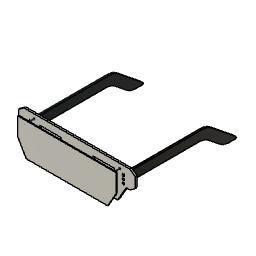
HyperShades mk.2 (Autodesk Fusion 360 design; units mm, degrees)
Autodesk Fusion 360 part; units mm, degrees
sketch "DiffSketch" plane through (0, 0, 0) normal (0, 1, 0) x (1, 0, 0)
  line L0 (-69.215, 0) -> (69.215, 0)
  line L1 (-69.215, 0) -> (-69.215, 25.4)
  line L2 (69.215, 0) -> (69.215, 25.4)
  line L3 (69.215, 25.4) -> (57.1899, 46.228)
  line L4 (57.1899, 46.228) -> (-0.1294, 46.228)
  line L5 (-69.215, 25.4) -> (-57.1899, 46.228)
  line L6 (-57.1899, 46.228) -> (-0.1294, 46.228)
  dimension "d1" = 138.43
  dimension "d3" = 25.4
  dimension "d4" = 25.4
  dimension "d5" = 150
  dimension "d6" = 150
  dimension "d26" = 46.228
  constraint horizontal L0
  constraint coincident origin L0
  constraint perpendicular L0 L1
  constraint perpendicular L0 L2
  constraint coincident L0 origin
  constraint midpoint L0 origin
  constraint horizontal L4
  constraint horizontal L6
  measures "d1" distance of L0.start L0.end
  measures "d3" distance of L0.start L1.end
  measures "d4" distance of L0.end L2.end
  measures "d5" angle of L2 L3
  measures "d6" angle of L1 L5
  measures "d26" vertical distance of origin L4.end
extrude "Extrude1" add sketch "DiffSketch" along normal blind 1.27 makes body 1
sketch "StandSketch" plane through (0, 1.27, 0) normal (0, 1, 0) x (-1, 0, 0)
  line L0 (69.215, 0) -> (-69.215, 0)
  line L1 (-69.215, 0) -> (-69.215, -25.4)
  line L2 (-69.215, -25.4) -> (-57.1899, -46.228)
  line L3 (-57.1899, -46.228) -> (57.1899, -46.228)
  line L4 (57.1899, -46.228) -> (69.215, -25.4)
  line L5 (69.215, -25.4) -> (69.215, 0)
  circle A0 centre (-60.325, -6.35) radius 1.016
  line L6 (-69.215, 0) -> (-60.325, 0) construction
  line L7 (-60.325, 0) -> (-60.325, -6.35) construction
  line L8 (-60.325, -6.35) -> (-69.215, -6.35) construction
  line L9 (-69.215, -6.35) -> (-69.215, 0) construction
  line L10 (69.215, 0) -> (60.325, 0) construction
  line L11 (60.325, 0) -> (60.325, -6.35) construction
  line L12 (60.325, -6.35) -> (69.215, -6.35) construction
  line L13 (69.215, -6.35) -> (69.215, 0) construction
  circle A1 centre (60.325, -6.35) radius 1.016
  line L14 (0, -46.228) -> (-12.7, -46.228) construction
  line L15 (-12.7, -46.228) -> (-12.7, -30.988) construction
  line L16 (-12.7, -30.988) -> (0, -30.988) construction
  line L17 (0, -30.988) -> (0, -46.228) construction
  line L18 (0, -46.228) -> (12.7, -46.228) construction
  line L19 (12.7, -46.228) -> (12.7, -30.988) construction
  line L20 (12.7, -30.988) -> (0, -30.988) construction
  line L21 (0, -30.988) -> (0, -46.228) construction
  circle A2 centre (-12.7, -30.988) radius 1.016
  circle A3 centre (12.7, -30.988) radius 1.016
  dimension "d10" = 2.032
  dimension "d11" = 8.89
  dimension "d12" = 6.35
  dimension "d23" = 8.89
  dimension "d24" = 6.35
  dimension "d25" = 2.032
  dimension "d27" = 12.7
  dimension "d28" = 15.24
  dimension "d29" = 12.7
  dimension "d30" = 15.24
  dimension "d31" = 2.032
  dimension "d32" = 2.032
  constraint horizontal L6
  constraint vertical L7
  constraint horizontal L8
  constraint vertical L9
  constraint coincident L0.end L1.start
  constraint coincident A0.centre L7.end
  constraint horizontal L10
  constraint vertical L11
  constraint horizontal L12
  constraint vertical L13
  constraint coincident L0.start L5.end
  constraint coincident L11.end L12.start
  constraint horizontal L14
  constraint vertical L15
  constraint horizontal L16
  constraint vertical L17
  constraint midpoint L3 L14.start
  constraint horizontal L18
  constraint vertical L19
  constraint horizontal L20
  constraint vertical L21
  constraint coincident L15.end L16.start
  constraint coincident L19.end L20.start
  measures "d10" diameter of A0
  measures "d11" distance of L0.end L6.end
  measures "d12" distance of L0.end L8.end
  measures "d23" distance of L0.start L10.end
  measures "d24" distance of L0.start L12.end
  measures "d25" diameter of A1
  measures "d27" distance of L14.start L14.end
  measures "d28" distance of L14.start L16.end
  measures "d29" distance of L14.start L18.end
  measures "d30" distance of L14.start L16.end
  measures "d31" diameter of A2
  measures "d32" diameter of A3
extrude "Extrude2" add sketch "StandSketch" along normal blind 12.7 separate body contours A0 | A1 | A2 | A3 makes body 2 at (60.3503, 9.7367, -5.3343) makes body 3 at (-60.2997, 9.7367, -5.3343) makes body 4 at (13.4783, 9.7367, -31.6411) makes body 5 at (-11.9217, 9.7367, -31.6411)
sketch "GlassSketch" plane through (0, 13.97, 0) normal (0, 1, 0) x (-1, 0, 0)
  circle A0 centre (-60.325, -6.35) radius 1.016
  line L0 (69.215, 0) -> (-69.215, 0)
  line L1 (-69.215, 0) -> (-69.215, -25.4)
  line L2 (-69.215, -25.4) -> (-57.1899, -46.228)
  line L3 (-57.1899, -46.228) -> (57.1899, -46.228)
  line L4 (57.1899, -46.228) -> (69.215, -25.4)
  line L5 (69.215, -25.4) -> (69.215, 0)
  line L6 (-12.7, -46.228) -> (12.7, -46.228)
  line L7 (-11.4475, -42.9716) -> (-3.556, -22.4537)
  line L8 (3.556, -22.4537) -> (11.4475, -42.9716)
  arc A1 (3.556, -22.4537) -> (-3.556, -22.4537) centre (0, -23.8214) ccw
  circle A2 centre (-12.7, -30.988) radius 1.016
  circle A3 centre (12.7, -30.988) radius 1.016
  circle A4 centre (60.325, -6.35) radius 1.016
  line L9 (16.1889, -46.228) -> (57.1899, -46.228)
  line L10 (-16.1889, -46.228) -> (-57.1899, -46.228)
  arc A5 (-16.1889, -46.228) -> (-11.4475, -42.9716) centre (-16.1889, -41.148) ccw
  arc A6 (11.4475, -42.9716) -> (16.1889, -46.228) centre (16.1889, -41.148) ccw
  point P0 (0, -46.228)
  point P1 (0, -13.208)
  dimension "d15" = 25.4
  dimension "d17" = 33.02
  dimension "d20" = 3.81
  dimension "d97" = 5.08
  dimension "d98" = 5.08
  constraint coincident L3 L6.start
  constraint parallel L3 L6
  constraint coincident L6 P0
  constraint midpoint L6 P0
  constraint vertical origin P0
  constraint vertical origin P1
  constraint coincident P1 L8
  constraint coincident P1 L7
  constraint tangent L8 A1
  constraint tangent L7 A1
  constraint coincident L3.end L4.start
  constraint coincident L2.end L3.start
  constraint coincident L6.start L10
  constraint coincident L6.start L7
  constraint tangent L10 A5
  constraint tangent L7 A5
  constraint coincident L6.end L8
  constraint coincident L6.end L9
  constraint tangent L8 A6
  constraint tangent L9 A6
  measures "d15" distance of L6.start L6.end
  measures "d17" vertical distance of L6.end P1
  measures "d20" radius of A1
  measures "d97" radius of A5
  measures "d98" radius of A6
extrude "Extrude4" add sketch "GlassSketch" along normal blind 2.54 separate body contours L0 L1 L2 L3 L4 L5 L7 L8 A1 L9 L10 A5 A6 makes body 6
sketch "EarSketch" plane through (69.215, 0, 0) normal (1, 0, 0) x (0, 1, 0)
  line L0 (13.97, 0) -> (13.97, -25.4)
  line L1 (13.97, -25.4) -> (16.51, -25.4)
  line L2 (16.51, -25.4) -> (16.51, 0)
  line L3 (16.51, 0) -> (13.97, 0)
  line L4 (16.51, -10.4595) -> (123.1933, -10.4595)
  line L5 (16.51, -23.1595) -> (118.7129, -23.1595)
  line L6 (16.51, -10.4595) -> (16.51, -12.9995)
  line L7 (16.51, -12.9995) -> (25.4, -12.9995)
  line L8 (25.4, -12.9995) -> (25.4, -15.5395)
  line L9 (25.4, -15.5395) -> (16.51, -15.5395)
  line L10 (16.51, -15.5395) -> (16.51, -18.0795)
  line L11 (16.51, -18.0795) -> (25.4, -18.0795)
  line L12 (25.4, -18.0795) -> (25.4, -20.6195)
  line L13 (25.4, -20.6195) -> (16.51, -20.6195)
  line L14 (16.51, -20.6195) -> (16.51, -23.1595)
  line L15 (16.51, 0) -> (170.18, 0) construction
  line L16 (136.7406, -15.2388) -> (170.9769, -42.8289)
  line L17 (132.2602, -27.9388) -> (147.6096, -40.3085)
  line L18 (161.1569, -45.0878) -> (170.18, -45.0878)
  arc A0 (132.2602, -27.9388) -> (118.7129, -23.1595) centre (118.7129, -44.7495) ccw
  arc A1 (136.7406, -15.2388) -> (123.1933, -10.4595) centre (123.1933, -32.0495) ccw
  arc A2 (170.18, -45.0878) -> (170.9769, -42.8289) centre (170.18, -43.8178) ccw
  arc A3 (147.6096, -40.3085) -> (161.1569, -45.0878) centre (161.1569, -23.4978) ccw
  point P0 (130.81, -10.4595)
  point P1 (16.51, -46.228)
  dimension "d44" = 12.7
  dimension "d45" = 2.54
  dimension "d51" = 114.3
  dimension "d52" = 153.67
  dimension "d55" = 12.7
  dimension "d56" = 8.89
  dimension "d57" = 12.7
  dimension "d62" = 21.59
  dimension "d63" = 21.59
  dimension "d64" = 1.27
  dimension "d65" = 21.59
  constraint coincident L2 L4.start
  constraint perpendicular L4 L6
  constraint perpendicular L6 L7
  constraint perpendicular L7 L8
  constraint horizontal L9
  constraint perpendicular L9 L10
  constraint perpendicular L8 L11
  constraint perpendicular L11 L12
  constraint coincident L2.end L3.start
  constraint perpendicular L2 L15
  constraint parallel L5 L18
  constraint parallel L16 L17
  constraint horizontal L13
  constraint equal L6 L8
  constraint equal L8 L10
  constraint equal L6 L12
  constraint equal L6 L14
  constraint equal L7 L9
  constraint equal L11 L13
  constraint equal L9 L11
  constraint tangent L5 A0
  constraint tangent L17 A0
  constraint coincident P0 L4
  constraint coincident P0 L16
  constraint tangent L4 A1
  constraint tangent L16 A1
  constraint tangent L16 A2
  constraint tangent L18 A2
  constraint tangent L17 A3
  constraint tangent L18 A3
  constraint vertical L15.end A2.centre
  measures "d44" distance of L4.start L5.start
  measures "d45" distance of L4.start L6.end
  measures "d51" distance of L4.start P0
  measures "d52" distance of L2.end L15.end
  measures "d55" distance of L16 L17
  measures "d56" distance of L6.end L7.end
  measures "d57" distance of L4 L5
  measures "d62" radius of A0
  measures "d63" radius of A1
  measures "d64" radius of A2
  measures "d65" radius of A3
extrude "Extrude7" add sketch "EarSketch" against normal blind 2.54 separate body contours L2 L4 L5 L6 L7 L8 L9 L10 L11 L12 L13 L14 L16 L17 L18 A0 A1 A2 A3 makes body 7
move_body "Move2" bodies 7 to x (1, 0, 0) y (0, 1, 0) z (0, 0, 1) at (-2.54, 0, 0)
extrude "Extrude8" cut 1 faces at (64.9817, 16.51, -12.1528) along direction (0, -1, 0) blind 7.62 on bodies 7 bodies 6
extrude "Extrude9" cut 1 faces at (64.9817, 16.51, -17.2328) along direction (0, -1, 0) blind 7.62 on bodies 7 bodies 6
extrude "Extrude10" cut 1 faces at (64.9817, 16.51, -22.3128) along direction (0, -1, 0) blind 10.16 on bodies 7 bodies 6
move_body "Move3" bodies 7 to x (1, 0, 0) y (0, 1, 0) z (0, 0, 1) at (-133.35, 0, -2.2405)
move_body "Move4" bodies 7 to x (1, 0, 0) y (0, 1, 0) z (0, 0, 1) at (2.54, 0, 2.54)
extrude "Extrude11" cut 1 faces at (-65.8283, 16.51, -11.8533) along direction (0, -1, 0) blind 12.7 on bodies 7 bodies 6
extrude "Extrude12" cut 1 faces at (-65.8283, 16.51, -16.9333) along direction (0, -1, 0) blind 10.16 on bodies 7 bodies 6
extrude "Extrude13" cut 1 faces at (-65.8283, 16.51, -22.0133) along direction (0, -1, 0) blind 15.24 on bodies 7 bodies 6
sketch "EyeHoleSketch" plane through (0, 16.51, 0) normal (0, 1, 0) x (-1, 0, 0)
  line L0 (66.675, -22.86) -> (64.135, -22.86)
  line L1 (64.135, -22.86) -> (64.135, -20.32)
  line L2 (64.135, -20.32) -> (66.675, -20.32)
  line L3 (66.675, -20.32) -> (66.675, -22.86)
  line L4 (66.675, -17.78) -> (64.135, -17.78)
  line L5 (64.135, -17.78) -> (64.135, -15.24)
  line L6 (64.135, -15.24) -> (66.675, -15.24)
  line L7 (66.675, -15.24) -> (66.675, -17.78)
  line L8 (66.675, -12.7) -> (64.135, -12.7)
  line L9 (64.135, -12.7) -> (64.135, -10.16)
  line L10 (64.135, -10.16) -> (66.675, -10.16)
  line L11 (66.675, -10.16) -> (66.675, -12.7)
  line L12 (-64.135, -23.1595) -> (-66.675, -23.1595)
  line L13 (-66.675, -23.1595) -> (-66.675, -20.6195)
  line L14 (-66.675, -20.6195) -> (-64.135, -20.6195)
  line L15 (-64.135, -20.6195) -> (-64.135, -23.1595)
  line L16 (-64.135, -18.0795) -> (-66.675, -18.0795)
  line L17 (-66.675, -18.0795) -> (-66.675, -15.5395)
  line L18 (-66.675, -15.5395) -> (-64.135, -15.5395)
  line L19 (-64.135, -15.5395) -> (-64.135, -18.0795)
  line L20 (-64.135, -12.9995) -> (-66.675, -12.9995)
  line L21 (-66.675, -12.9995) -> (-66.675, -10.4595)
  line L22 (-66.675, -10.4595) -> (-64.135, -10.4595)
  line L23 (-64.135, -10.4595) -> (-64.135, -12.9995)
  circle A0 centre (60.325, -6.35) radius 1.016
  circle A1 centre (12.7, -30.988) radius 1.016
  circle A2 centre (-12.7, -30.988) radius 1.016
  circle A3 centre (-60.325, -6.35) radius 1.016
  line L24 (16.1889, -46.228) -> (57.1899, -46.228)
  line L25 (57.1899, -46.228) -> (69.215, -25.4)
  line L26 (69.215, -25.4) -> (69.215, 0)
  line L27 (69.215, 0) -> (-69.215, 0)
  line L28 (-69.215, 0) -> (-69.215, -25.4)
  line L29 (-69.215, -25.4) -> (-57.1899, -46.228)
  line L30 (0, -10) -> (30, -10) construction
  line L31 (22.38, -10) -> (52.38, -10)
  line L32 (22.38, -10) -> (22.38, -25)
  line L33 (52.38, -10) -> (52.38, -25)
  line L34 (52.38, -25) -> (48.88, -31.0622)
  line L35 (22.38, -25) -> (25.88, -31.0622)
  line L36 (25.88, -31.0622) -> (48.88, -31.0622)
  line L37 (0, 0) -> (0, 13.9322) construction
  line L38 (-22.38, -10) -> (-52.38, -10)
  line L39 (-22.38, -10) -> (-22.38, -25)
  line L40 (-25.88, -31.0622) -> (-48.88, -31.0622)
  line L41 (-22.38, -25) -> (-25.88, -31.0622)
  line L42 (-52.38, -10) -> (-52.38, -25)
  line L43 (-52.38, -25) -> (-48.88, -31.0622)
  line L44 (3.556, -22.4537) -> (11.4475, -42.9716)
  arc A4 (11.4475, -42.9716) -> (16.1889, -46.228) centre (16.1889, -41.148) ccw
  line L45 (-57.1899, -46.228) -> (-16.1889, -46.228)
  arc A5 (-16.1889, -46.228) -> (-11.4475, -42.9716) centre (-16.1889, -41.148) ccw
  line L46 (-11.4475, -42.9716) -> (-3.556, -22.4537)
  arc A6 (3.556, -22.4537) -> (-3.556, -22.4537) centre (0, -23.8214) ccw
  dimension "d78" = 30
  dimension "d79" = 30
  dimension "d80" = 7.62
  dimension "d81" = 10
  dimension "d82" = 15
  dimension "d83" = 7
  dimension "d84" = 7
  dimension "d85" = 150
  constraint parallel L27 L30
  constraint coincident L30 L31.start
  constraint parallel L30 L31
  constraint vertical L37.start L30.start
  constraint perpendicular L30 L32
  constraint perpendicular L31 L33
  constraint horizontal L34.end L35.end
  constraint equal L32 L33
  constraint coincident L37.start origin
  constraint perpendicular L27 L37
  constraint symmetric L31.start L37 L38.start
  constraint symmetric L31.end L37 L38.end
  constraint symmetric L32.end L37 L39.end
  constraint symmetric L33.end L37 L42.end
  constraint symmetric L34.end L37 L40.end
  constraint symmetric L35.end L37 L40.start
  measures "d78" distance of L30.start L30.end
  measures "d79" distance of L31.start L31.end
  measures "d80" distance of L30.end L31.start
  measures "d81" distance of L37.start L30.start
  measures "d82" distance of L31.start L32.end
  measures "d83" distance of L33.end L34.end
  measures "d84" distance of L32.end L35.end
  measures "d85" angle of L32 L35
extrude "Extrude14" cut sketch "EyeHoleSketch" against normal up to surface (2.54 mm away) contours L31 L32 L33 L34 L35 L36 | L38 L39 L40 L41 L42 L43 bodies 6
sketch "Sketch7" plane through (0, 16.51, 0) normal (0, 1, 0) x (-1, 0, 0)
  line L0 (-22.38, -25) -> (-25.88, -31.0622)
  line L1 (-25.88, -31.0622) -> (-48.88, -31.0622)
  line L2 (-48.88, -31.0622) -> (-52.38, -25)
  line L3 (-52.38, -25) -> (-52.38, -10)
  line L4 (-52.38, -10) -> (-22.38, -10)
  line L5 (-22.38, -10) -> (-22.38, -25)
  line L6 (52.38, -10) -> (52.38, -25)
  line L7 (52.38, -25) -> (48.88, -31.0622)
  line L8 (48.88, -31.0622) -> (25.88, -31.0622)
  line L9 (25.88, -31.0622) -> (22.38, -25)
  line L10 (22.38, -25) -> (22.38, -10)
  line L11 (22.38, -10) -> (52.38, -10)
  line L12 (66.675, -22.86) -> (64.135, -22.86)
  line L13 (64.135, -22.86) -> (64.135, -20.32)
  line L14 (64.135, -20.32) -> (66.675, -20.32)
  line L15 (66.675, -20.32) -> (66.675, -22.86)
  line L16 (66.675, -17.78) -> (64.135, -17.78)
  line L17 (64.135, -17.78) -> (64.135, -15.24)
  line L18 (64.135, -15.24) -> (66.675, -15.24)
  line L19 (66.675, -15.24) -> (66.675, -17.78)
  line L20 (66.675, -12.7) -> (64.135, -12.7)
  line L21 (64.135, -12.7) -> (64.135, -10.16)
  line L22 (64.135, -10.16) -> (66.675, -10.16)
  line L23 (66.675, -10.16) -> (66.675, -12.7)
  line L24 (-64.135, -23.1595) -> (-66.675, -23.1595)
  line L25 (-66.675, -23.1595) -> (-66.675, -20.6195)
  line L26 (-66.675, -20.6195) -> (-64.135, -20.6195)
  line L27 (-64.135, -20.6195) -> (-64.135, -23.1595)
  line L28 (-64.135, -18.0795) -> (-66.675, -18.0795)
  line L29 (-66.675, -18.0795) -> (-66.675, -15.5395)
  line L30 (-66.675, -15.5395) -> (-64.135, -15.5395)
  line L31 (-64.135, -15.5395) -> (-64.135, -18.0795)
  line L32 (-64.135, -12.9995) -> (-66.675, -12.9995)
  line L33 (-66.675, -12.9995) -> (-66.675, -10.4595)
  line L34 (-66.675, -10.4595) -> (-64.135, -10.4595)
  line L35 (-64.135, -10.4595) -> (-64.135, -12.9995)
  circle A0 centre (60.325, -6.35) radius 1.016
  circle A1 centre (12.7, -30.988) radius 1.016
  circle A2 centre (-12.7, -30.988) radius 1.016
  circle A3 centre (-60.325, -6.35) radius 1.016
  line L36 (16.1889, -46.228) -> (57.1899, -46.228)
  line L37 (57.1899, -46.228) -> (69.215, -25.4)
  line L38 (69.215, -25.4) -> (69.215, 0)
  line L39 (69.215, 0) -> (-69.215, 0)
  line L40 (-69.215, 0) -> (-69.215, -25.4)
  line L41 (-69.215, -25.4) -> (-57.1899, -46.228)
  line L42 (3.556, -22.4537) -> (11.4475, -42.9716)
  arc A4 (11.4475, -42.9716) -> (16.1889, -46.228) centre (16.1889, -41.148) ccw
  line L43 (-57.1899, -46.228) -> (-16.1889, -46.228)
  arc A5 (-16.1889, -46.228) -> (-11.4475, -42.9716) centre (-16.1889, -41.148) ccw
  line L44 (-11.4475, -42.9716) -> (-3.556, -22.4537)
  arc A6 (3.556, -22.4537) -> (-3.556, -22.4537) centre (0, -23.8214) ccw
extrude "Extrude15" add sketch "Sketch7" against normal blind 1.27 contours L12 L13 L14 L15 | L16 L17 L18 L19 | L20 L21 L22 L23 bodies 7
sketch "Sketch9" plane through (-64.135, 0, 0) normal (1, 0, 0) x (0, 1, 0)
  line L0 (15.24, -22.86) -> (118.7129, -22.86)
  arc A0 (132.2602, -27.6393) -> (118.7129, -22.86) centre (118.7129, -44.45) ccw
  line L1 (132.2602, -27.6393) -> (147.6096, -40.009)
  arc A1 (147.6096, -40.009) -> (161.1569, -44.7883) centre (161.1569, -23.1983) ccw
  line L2 (161.1569, -44.7883) -> (170.18, -44.7883)
  arc A2 (170.18, -44.7883) -> (170.9769, -42.5294) centre (170.18, -43.5183) ccw
  line L3 (170.9769, -42.5294) -> (136.7406, -14.9393)
  arc A3 (136.7406, -14.9393) -> (123.1933, -10.16) centre (123.1933, -31.75) ccw
  line L4 (123.1933, -10.16) -> (15.24, -10.16)
  line L5 (15.24, -10.16) -> (15.24, -12.7)
  line L6 (15.24, -12.7) -> (25.4, -12.7)
  line L7 (25.4, -12.7) -> (25.4, -15.24)
  line L8 (25.4, -15.24) -> (15.24, -15.24)
  line L9 (15.24, -15.24) -> (15.24, -17.78)
  line L10 (15.24, -17.78) -> (25.4, -17.78)
  line L11 (25.4, -17.78) -> (25.4, -20.32)
  line L12 (25.4, -20.32) -> (15.24, -20.32)
  line L13 (15.24, -20.32) -> (15.24, -22.86)
sketch "Sketch10" plane through (0, 1.27, 0) normal (0, 1, 0) x (-1, 0, 0)
  line L0 (69.215, 0) -> (-69.215, 0)
  line L1 (-69.215, 0) -> (-69.215, -25.4)
  line L2 (-69.215, -25.4) -> (-57.1899, -46.228)
  line L3 (-57.1899, -46.228) -> (57.1899, -46.228)
  line L4 (57.1899, -46.228) -> (69.215, -25.4)
  line L5 (69.215, -25.4) -> (69.215, 0)
  circle A0 centre (-60.325, -6.35) radius 1.016
  circle A1 centre (-12.7, -30.988) radius 1.016
  circle A2 centre (12.7, -30.988) radius 1.016
  circle A3 centre (60.325, -6.35) radius 1.016
copy_body "CopyPasteBodies2" bodies 7 makes body 8
move_body "Move5" bodies 8 to x (1, 0, 0) y (0, 1, 0) z (0, 0, 1) at (130.81, 0, -0.2995)
sketch "Sketch11" plane through (0, 13.97, 0) normal (0, -1, 0) x (1, 0, 0)
  line L0 (25.88, -31.0622) -> (22.38, -25)
  line L1 (22.38, -25) -> (22.38, -10)
  line L2 (22.38, -10) -> (52.38, -10)
  line L3 (52.38, -10) -> (52.38, -25)
  line L4 (52.38, -25) -> (48.88, -31.0622)
  line L5 (48.88, -31.0622) -> (25.88, -31.0622)
  line L6 (-52.38, -25) -> (-52.38, -10)
  line L7 (-52.38, -10) -> (-22.38, -10)
  line L8 (-22.38, -10) -> (-22.38, -25)
  line L9 (-22.38, -25) -> (-25.88, -31.0622)
  line L10 (-25.88, -31.0622) -> (-48.88, -31.0622)
  line L11 (-48.88, -31.0622) -> (-52.38, -25)
  line L12 (-64.135, -22.86) -> (-66.675, -22.86)
  line L13 (-66.675, -22.86) -> (-66.675, -20.32)
  line L14 (-66.675, -20.32) -> (-64.135, -20.32)
  line L15 (-64.135, -20.32) -> (-64.135, -22.86)
  line L16 (-64.135, -17.78) -> (-66.675, -17.78)
  line L17 (-66.675, -17.78) -> (-66.675, -15.24)
  line L18 (-66.675, -15.24) -> (-64.135, -15.24)
  line L19 (-64.135, -15.24) -> (-64.135, -17.78)
  line L20 (-64.135, -12.7) -> (-66.675, -12.7)
  line L21 (-66.675, -12.7) -> (-66.675, -10.16)
  line L22 (-66.675, -10.16) -> (-64.135, -10.16)
  line L23 (-64.135, -10.16) -> (-64.135, -12.7)
  line L24 (66.675, -23.1595) -> (64.135, -23.1595)
  line L25 (64.135, -23.1595) -> (64.135, -20.6195)
  line L26 (64.135, -20.6195) -> (66.675, -20.6195)
  line L27 (66.675, -20.6195) -> (66.675, -23.1595)
  line L28 (66.675, -18.0795) -> (64.135, -18.0795)
  line L29 (64.135, -18.0795) -> (64.135, -15.5395)
  line L30 (64.135, -15.5395) -> (66.675, -15.5395)
  line L31 (66.675, -15.5395) -> (66.675, -18.0795)
  line L32 (66.675, -12.9995) -> (64.135, -12.9995)
  line L33 (64.135, -12.9995) -> (64.135, -10.4595)
  line L34 (64.135, -10.4595) -> (66.675, -10.4595)
  line L35 (66.675, -10.4595) -> (66.675, -12.9995)
  circle A0 centre (-60.325, -6.35) radius 1.016
  circle A1 centre (-12.7, -30.988) radius 1.016
  circle A2 centre (12.7, -30.988) radius 1.016
  circle A3 centre (60.325, -6.35) radius 1.016
  line L36 (-57.1899, -46.228) -> (-16.1889, -46.228)
  line L37 (57.1899, -46.228) -> (69.215, -25.4)
  line L38 (69.215, -25.4) -> (69.215, 0)
  line L39 (69.215, 0) -> (-69.215, 0)
  line L40 (-69.215, 0) -> (-69.215, -25.4)
  line L41 (-69.215, -25.4) -> (-57.1899, -46.228)
  line L42 (69.215, 0) -> (74.295, 0)
  line L43 (69.215, -25.4) -> (74.295, -25.4)
  line L44 (0, 0) -> (0, -20.0114) construction
  line L45 (74.295, -25.4) -> (81.915, -20.0644)
  line L46 (81.915, -20.0644) -> (81.915, -5.3356)
  line L47 (81.915, -5.3356) -> (74.295, 0)
  line L48 (-69.215, 0) -> (-74.295, 0)
  line L49 (-81.915, -5.3356) -> (-74.295, 0)
  line L50 (-81.915, -20.0644) -> (-81.915, -5.3356)
  line L51 (-74.295, -25.4) -> (-81.915, -20.0644)
  line L52 (-69.215, -25.4) -> (-74.295, -25.4)
  line L53 (-11.4475, -42.9716) -> (-3.556, -22.4537)
  arc A4 (3.556, -22.4537) -> (-3.556, -22.4537) centre (0, -23.8214) ccw
  line L54 (3.556, -22.4537) -> (11.4475, -42.9716)
  arc A5 (11.4475, -42.9716) -> (16.1889, -46.228) centre (16.1889, -41.148) ccw
  line L55 (16.1889, -46.228) -> (57.1899, -46.228)
  arc A6 (-16.1889, -46.228) -> (-11.4475, -42.9716) centre (-16.1889, -41.148) ccw
  dimension "d90" = 5.08
  dimension "d91" = 5.08
  dimension "d92" = 145
  dimension "d93" = 145
  dimension "d94" = 12.7
  constraint coincident L38.end L39.start
  constraint perpendicular L38 L42
  constraint coincident L37.end L38.start
  constraint perpendicular L38 L43
  constraint coincident L44.start origin
  constraint perpendicular L43 L46
  constraint symmetric L38.end L44 L39.end
  constraint symmetric L42.end L44 L48.end
  constraint symmetric L37.end L44 L40.end
  constraint symmetric L43.end L44 L51.start
  constraint symmetric L44 L45.end L50.start
  constraint symmetric L44 L46.end L49.start
  measures "d90" distance of L38.end L42.end
  measures "d91" distance of L37.end L43.end
  measures "d92" angle of L42 L47
  measures "d93" angle of L43 L45
  measures "d94" distance of L38 L46
extrude "Extrude16" add sketch "Sketch11" against normal up to surface (2.54 mm away) contours L40 L48 L49 L50 L51 L52 | L38 L42 L43 L45 L46 L47 bodies 6
sketch "Sketch12" plane through (0, 13.97, 0) normal (0, -1, 0) x (1, 0, 0)
  line L0 (25.88, -31.0622) -> (22.38, -25)
  line L1 (22.38, -25) -> (22.38, -10)
  line L2 (22.38, -10) -> (52.38, -10)
  line L3 (52.38, -10) -> (52.38, -25)
  line L4 (52.38, -25) -> (48.88, -31.0622)
  line L5 (48.88, -31.0622) -> (25.88, -31.0622)
  line L6 (-52.38, -25) -> (-52.38, -10)
  line L7 (-52.38, -10) -> (-22.38, -10)
  line L8 (-22.38, -10) -> (-22.38, -25)
  line L9 (-22.38, -25) -> (-25.88, -31.0622)
  line L10 (-25.88, -31.0622) -> (-48.88, -31.0622)
  line L11 (-48.88, -31.0622) -> (-52.38, -25)
  line L12 (-64.135, -22.86) -> (-66.675, -22.86)
  line L13 (-66.675, -22.86) -> (-66.675, -20.32)
  line L14 (-66.675, -20.32) -> (-64.135, -20.32)
  line L15 (-64.135, -20.32) -> (-64.135, -22.86)
  line L16 (-64.135, -17.78) -> (-66.675, -17.78)
  line L17 (-66.675, -17.78) -> (-66.675, -15.24)
  line L18 (-66.675, -15.24) -> (-64.135, -15.24)
  line L19 (-64.135, -15.24) -> (-64.135, -17.78)
  line L20 (-64.135, -12.7) -> (-66.675, -12.7)
  line L21 (-66.675, -12.7) -> (-66.675, -10.16)
  line L22 (-66.675, -10.16) -> (-64.135, -10.16)
  line L23 (-64.135, -10.16) -> (-64.135, -12.7)
  line L24 (66.675, -23.1595) -> (64.135, -23.1595)
  line L25 (64.135, -23.1595) -> (64.135, -20.6195)
  line L26 (64.135, -20.6195) -> (66.675, -20.6195)
  line L27 (66.675, -20.6195) -> (66.675, -23.1595)
  line L28 (66.675, -18.0795) -> (64.135, -18.0795)
  line L29 (64.135, -18.0795) -> (64.135, -15.5395)
  line L30 (64.135, -15.5395) -> (66.675, -15.5395)
  line L31 (66.675, -15.5395) -> (66.675, -18.0795)
  line L32 (66.675, -12.9995) -> (64.135, -12.9995)
  line L33 (64.135, -12.9995) -> (64.135, -10.4595)
  line L34 (64.135, -10.4595) -> (66.675, -10.4595)
  line L35 (66.675, -10.4595) -> (66.675, -12.9995)
  circle A0 centre (60.325, -6.35) radius 1.016
  circle A1 centre (12.7, -30.988) radius 1.016
  circle A2 centre (-12.7, -30.988) radius 1.016
  circle A3 centre (-60.325, -6.35) radius 1.016
  line L36 (-11.4475, -42.9716) -> (-3.556, -22.4537)
  arc A4 (3.556, -22.4537) -> (-3.556, -22.4537) centre (0, -23.8214) ccw
  line L37 (3.556, -22.4537) -> (11.4475, -42.9716)
  arc A5 (11.4475, -42.9716) -> (16.1889, -46.228) centre (16.1889, -41.148) ccw
  line L38 (16.1889, -46.228) -> (57.1899, -46.228)
  line L39 (57.1899, -46.228) -> (69.215, -25.4)
  line L40 (69.215, -25.4) -> (74.295, -25.4)
  line L41 (74.295, -25.4) -> (81.915, -20.0644)
  line L42 (81.915, -20.0644) -> (81.915, -5.3356)
  line L43 (81.915, -5.3356) -> (74.295, 0)
  line L44 (74.295, 0) -> (-74.295, 0)
  line L45 (-74.295, 0) -> (-81.915, -5.3356)
  line L46 (-81.915, -5.3356) -> (-81.915, -20.0644)
  line L47 (-81.915, -20.0644) -> (-74.295, -25.4)
  line L48 (-74.295, -25.4) -> (-69.215, -25.4)
  line L49 (-69.215, -25.4) -> (-57.1899, -46.228)
  line L50 (-57.1899, -46.228) -> (-16.1889, -46.228)
  arc A6 (-16.1889, -46.228) -> (-11.4475, -42.9716) centre (-16.1889, -41.148) ccw
sketch "Sketch13" plane through (-66.675, 0, 0) normal (-1, 0, 0) x (0, -1, 0)
  line L0 (-15.24, -20.32) -> (-25.4, -20.32)
  line L1 (-25.4, -20.32) -> (-25.4, -17.78)
  line L2 (-25.4, -17.78) -> (-15.24, -17.78)
  line L3 (-15.24, -17.78) -> (-15.24, -15.24)
  line L4 (-15.24, -15.24) -> (-25.4, -15.24)
  line L5 (-25.4, -15.24) -> (-25.4, -12.7)
  line L6 (-25.4, -12.7) -> (-15.24, -12.7)
  line L7 (-15.24, -12.7) -> (-15.24, -10.16)
  line L8 (-15.24, -10.16) -> (-123.1933, -10.16)
  arc A0 (-123.1933, -10.16) -> (-136.7406, -14.9393) centre (-123.1933, -31.75) ccw
  line L9 (-136.7406, -14.9393) -> (-170.9769, -42.5294)
  arc A1 (-170.9769, -42.5294) -> (-170.18, -44.7883) centre (-170.18, -43.5183) ccw
  line L10 (-170.18, -44.7883) -> (-161.1569, -44.7883)
  arc A2 (-161.1569, -44.7883) -> (-147.6096, -40.009) centre (-161.1569, -23.1983) ccw
  line L11 (-147.6096, -40.009) -> (-132.2602, -27.6393)
  arc A3 (-118.7129, -22.86) -> (-132.2602, -27.6393) centre (-118.7129, -44.45) ccw
  line L12 (-118.7129, -22.86) -> (-15.24, -22.86)
  line L13 (-15.24, -22.86) -> (-15.24, -20.32)
equation "d21 = matThickness"
equation "matThickness = 0.1 in"
equation "d60 = -matThickness"
named bodies: "Diffuser", "Standoff", "Glasses", "Standoff(1)", "Standoff(2)", "Standoff(3)", "Ear Piece", "Ear Piece (1)"
